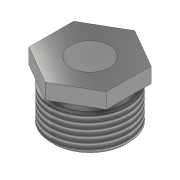
# Autodesk Inventor part: 螺套
Saved by Autodesk Inventor 2022 (Build 260153000, 153)
## iProperties
Created: 2023-03-14
Part Number: 螺套
Material: 不锈钢
Document SubType Name: Modeling
Designer: Lzy18
Density: 8 g/cm^3
Appearance: 半抛光
Author: Lzy18
Autodesk Inventor part; units mm, degrees
ref_plane "YZ Plane" through (0, 0, 0) normal (1, 0, 0) x (0, 1, 0)
ref_plane "XZ Plane" through (0, 0, 0) normal (0, 1, 0) x (-1, 0, 0)
ref_plane "XY Plane" through (0, 0, 0) normal (0, 0, 1) x (1, 0, 0)
sketch "草图1" plane through (0, 0, 0) normal (0, 1, 0) x (-1, 0, 0)
  line L0 (20, -11.547) -> (0, -23.094)
  line L1 (0, -23.094) -> (-20, -11.547)
  line L2 (-20, -11.547) -> (-20, 11.547)
  line L3 (-20, 11.547) -> (0, 23.094)
  line L4 (0, 23.094) -> (20, 11.547)
  line L5 (20, 11.547) -> (20, -11.547)
  point P0 (0, 0)
  point P1 (0, 0)
  dimension "d0" = 40
  constraints: 12 end point, 1 coincident, 13 other
  measures "d0" distance between parallel lines of L2 L5
extrude "拉伸1" add sketch "草图1" along normal mid plane 8
sketch "草图4" plane through (0, -4, 0) normal (0, -1, 0) x (1, 0, 0)
  circle A0 centre (0, 0) radius 18
  dimension "d18" = 36
  constraints: 1 centre point, 1 coincident
  measures "d18" diameter of A0
extrude "拉伸3" add sketch "草图4" along normal blind 4
sketch "草图5" plane through (0, -8, 0) normal (0, -1, 0) x (1, 0, 0)
  circle A0 centre (0, 0) radius 20
  dimension "d21" = 40
  constraints: 1 centre point, 1 coincident
  measures "d21" diameter of A0
extrude "拉伸4" add sketch "草图5" along normal blind 18
thread "螺纹1" size "M40x3" class "6g" standard "GB Metric profile" full length
sketch "草图6" plane through (0, 0, 0) normal (0, 0, 1) x (1, 0, 0)
  line L0 (0, 4) -> (20, 4) projected
  line L1 (-20, -26) -> (20, -26) projected
  line L2 (0, 11.1674) -> (0, -43.9009)
  line L3 (10, -22.5359) -> (16, -26)
  line L4 (10, 4) -> (10, -22.5359)
  line L5 (20, -4) -> (20, 4) projected
  line L6 (0, 4) -> (20, 4) projected
  line L7 (0, -4) -> (0, 4) projected
  line L8 (20, -4) -> (0, -4) projected
  line L9 (-20, -26) -> (20, -26) projected
  line L10 (-20, -8) -> (20, -8) projected
  point P0 (0, 0)
  point P1 (0, -26)
  dimension "d28" = 60
  dimension "d29" = 16
  constraints: 6 end point, 2 point on line, 2 vertical, 1 midpoint
  measures "d28" angle of L2 L3
  measures "d29" distance from line of L2 L3.end
revolve "旋转2" cut sketch "草图6" angle 360 about axis through (0, 11.1674, 0) along (0, -1, 0) contours L0 L4 L8 L2 | L8 L4 L10 L2 | L10 L4 L3 L1 L2
chamfer "倒角2" distance 1.5 angle 45 1 edges at (-20, -26, 0)
